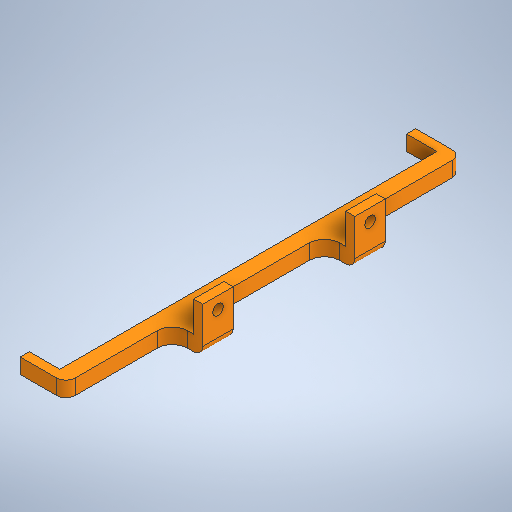
# Autodesk Inventor part: pare-chocs
Saved by Autodesk Inventor 2025 (Build 290162000, 162)
## iProperties
Created: 2024-10-10
Part Number: pare-chocs
Material: Générique
Document SubType Name: Modeling
Designer: chass
Density: 1 g/cm^3
Appearance: Par défaut
Author: chass
Autodesk Inventor part; units mm, degrees
ref_plane "YZ Plane" through (0, 0, 0) normal (1, 0, 0) x (0, 1, 0)
ref_plane "XZ Plane" through (0, 0, 0) normal (0, 1, 0) x (-1, 0, 0)
ref_plane "XY Plane" through (0, 0, 0) normal (0, 0, 1) x (1, 0, 0)
sketch "Esquisse1" plane through (0, 0, 0) normal (1, 0, 0) x (0, 1, 0)
  line L0 (-2.5, 65) -> (2.5, 65)
  line L1 (2.5, 65) -> (2.5, -65)
  line L2 (2.5, -65) -> (-2.5, -65)
  line L3 (-2.5, -65) -> (-2.5, 65)
  line L4 (2.5, 65) -> (-2.5, -65)
  line L5 (2.5, -65) -> (-2.5, 65)
  point P0 (0, 0)
  point P1 (0, 0)
  point P2 (0, 0)
  dimension "d0" = 130
  dimension "d1" = 5
  constraints: 12 end point, 2 midpoint, 2 parallel, 1 coincident, 1 horizontal, 1 perpendicular
  measures "d0" distance of L0.end L1.end
  measures "d1" distance of L1.end L2.end
extrude "Extrusion1" add sketch "Esquisse1" along normal blind 5
sketch "Esquisse2" plane through (5, 0, 0) normal (1, 0, 0) x (0, 0, -1)
  line L0 (65, 2.5) -> (-65, 2.5) projected
  line L1 (-65, -2.5) -> (65, -2.5) projected
  line L2 (-30, 2.5) -> (-20, 2.5)
  line L3 (-20, 2.5) -> (-20, -2.5)
  line L4 (-20, -2.5) -> (-30, -2.5)
  line L5 (-30, -2.5) -> (-30, 2.5)
  line L6 (0, 13) -> (0, -16)
  line L7 (30, 2.5) -> (20, 2.5)
  line L8 (20, 2.5) -> (20, -2.5)
  line L9 (20, -2.5) -> (30, -2.5)
  line L10 (30, -2.5) -> (30, 2.5)
  point P0 (0, 0)
  point P1 (-20, 2.5)
  point P2 (30, -2.5)
  point P3 (30, 2.5)
  point P4 (20, 2.5)
  point P5 (20, -2.5)
  dimension "d4" = 10
  dimension "d5" = 20
  constraints: 18 end point, 4 symmetric about line, 3 point on line, 2 parallel, 1 horizontal, 1 perpendicular, 1 vertical
  measures "d4" distance between parallel lines of L3 L5
  measures "d5" distance between parallel lines of L3 L6
extrude "Extrusion2" add sketch "Esquisse2" along normal blind 10 contours L10 L1 L8 L0 | L3 L1 L5 L0
sketch "Esquisse3" plane through (0, 2.5, 65) normal (0, 1, 0) x (1, 0, 0)
  line L0 (15, 45) -> (15, 35) projected
  line L1 (5, 45) -> (15, 45) projected
  line L2 (15, 35) -> (12, 35)
  line L3 (12, 35) -> (12, 45)
  line L4 (12, 45) -> (15, 45)
  line L5 (15, 45) -> (15, 35)
  line L6 (-9, 65) -> (24, 65)
  line L7 (15, 85) -> (15, 95)
  line L8 (15, 95) -> (12, 95)
  line L9 (12, 95) -> (12, 85)
  line L10 (12, 85) -> (15, 85)
  line L11 (15, 85) -> (15, 95)
  point P0 (0, 65)
  constraints: 20 end point, 5 symmetric about line, 2 horizontal, 2 parallel, 1 perpendicular, 1 point on line
extrude "Extrusion3" add sketch "Esquisse3" along normal blind 10
sketch "Esquisse4" plane through (15, 0, 0) normal (1, 0, 0) x (0, 0, -1)
  circle A0 centre (-25, 8.5) radius 1.75
  line L0 (0, 20) -> (0, -21)
  circle A1 centre (25, 8.5) radius 1.75
  line L1 (-30, 12.5) -> (-20, 12.5) projected
  line L2 (-20, -2.5) -> (-20, 12.5) projected
  point P0 (0, 0)
  dimension "d10" = 3.5
  dimension "d11" = 4
  dimension "d19" = 5
  constraints: 2 centre point, 2 end point, 1 symmetric about line, 1 vertical, 1 other
  measures "d10" diameter of A0
  measures "d11" distance from line of L1 A0.centre
  measures "d19" distance from line of L2 A0.centre
extrude "Extrusion4" cut sketch "Esquisse4" against normal blind 10
fillet "Congé1" radius 5 4 edges at (5, 0, 30) (5, 0, -20) (5, 0, 20) (5, 0, -30)
fillet "Congé2" radius 3 2 edges at (15, -2.5, 25) (15, -2.5, -25)
fillet "Congé3" radius 3 2 edges at (5, 0, -65) (5, 0, 65)
sketch "Esquisse5" plane through (0, 0, 0) normal (-1, 0, 0) x (0, 0, 1)
  line L0 (-65, 2.5) -> (65, 2.5) projected
  line L1 (65, -2.5) -> (-65, -2.5) projected
  line L2 (-65, 2.5) -> (-62, 2.5)
  line L3 (-62, 2.5) -> (-62, -2.5)
  line L4 (-62, -2.5) -> (-65, -2.5)
  line L5 (-65, -2.5) -> (-65, 2.5)
  line L6 (0, 19) -> (0, -21)
  line L7 (65, 2.5) -> (62, 2.5)
  line L8 (62, 2.5) -> (62, -2.5)
  line L9 (62, -2.5) -> (65, -2.5)
  line L10 (65, -2.5) -> (65, 2.5)
  point P0 (0, 0)
  point P1 (65, -2.5)
  constraints: 18 end point, 4 symmetric about line, 2 parallel, 1 horizontal, 1 perpendicular, 1 point on line, 1 vertical
extrude "Extrusion5" add sketch "Esquisse5" along normal blind 10 contours L0 L3 L1 L5 | L0 L10 L1 L8
